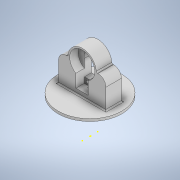
# Autodesk Inventor part: TAPA- 1
Saved by Autodesk Inventor 2021 (Build 250183000, 183)
## iProperties
Created: 2023-04-04
Part Number: TAPA- 1
Material: Generic
Document SubType Name: Modeling
Designer: PC
Density: 1 g/cm^3
Appearance: Default
Author: PC
Autodesk Inventor part; units mm, degrees
ref_plane "YZ Plane" through (0, 0, 0) normal (1, 0, 0) x (0, 1, 0)
ref_plane "XZ Plane" through (0, 0, 0) normal (0, 1, 0) x (-1, 0, 0)
sketch "Sketch1" plane through (0, 0, 0) normal (0, 1, 0) x (-1, 0, 0)
  point P0 (0, 0)
ref_plane "Work Plane26" through (0, 4, 0) normal (0, 1, 0) x (1, 0, 0)
ref_plane "Work Plane42" through (0, 54.25, 0) normal (0, 1, 0) x (-1, 0, 0)
sketch "Sketch7" plane through (0, 54.25, 0) normal (0, 1, 0) x (-1, 0, 0)
  circle A0 centre (0, 0) radius 50 projected
  circle A1 centre (0, 0) radius 52.5
  dimension "d12" = 105
  constraints: 1 centre point, 1 coincident
  measures "d12" diameter of A1
extrude "Extrusion5" add sketch "Sketch7" along normal blind 4 contours A0 | A1
ref_plane "Work Plane34" through (0, 58.25, 0) normal (0, 1, 0) x (1, 0, 0)
sketch "Sketch8" plane through (0, 58.25, 0) normal (0, 1, 0) x (1, 0, 0)
  circle A0 centre (0, 0) radius 51
  dimension "d15" = 102
  constraints: 1 centre point, 1 coincident
  measures "d15" diameter of A0
extrude "Extrusion6" cut sketch "Sketch8" against normal blind 4.5
ref_plane "Work Plane33" through (0, 58.25, 0) normal (0, 1, 0) x (1, 0, 0)
sketch "Sketch12" plane through (0, 58.25, 0) normal (0, 1, 0) x (1, 0, 0)
  circle A0 centre (0, 0) radius 52.5
  constraints: 1 centre point, 1 coincident
extrude "Extrusion7" add sketch "Sketch12" along normal blind 4
ref_plane "Work Plane30" through (0, 54.25, 0) normal (0, 1, 0) x (-1, 0, 0)
sketch "Sketch10" plane through (0, 54.25, 0) normal (0, 1, 0) x (-1, 0, 0)
  point P0 (0, 0)
ref_plane "Work Plane31" through (0, 54.25, 0) normal (0, 1, 0) x (-1, 0, 0)
sketch "Sketch11" plane through (0, 54.25, 0) normal (0, 1, 0) x (-1, 0, 0)
  point P0 (0, 0)
sketch "Sketch13" plane through (0, 62.25, 0) normal (0, 1, 0) x (1, 0, 0)
  point P0 (0, 0)
ref_plane "Work Plane35" through (0, 62.25, 0) normal (0, 1, 0) x (1, 0, 0)
sketch "Sketch18" plane through (0, 0, 0) normal (0, 1, 0) x (-1, 0, 0)
  point P0 (0, 0)
sketch "Sketch19" plane through (0, 0, 0) normal (0, 0, 1) x (1, 0, 0)
  point P0 (0, 0)
sketch "Sketch32" plane through (0, 62.25, 0) normal (0, 1, 0) x (1, 0, 0)
  point P0 (0, 0)
sketch "Sketch33" plane through (0, 62.25, 0) normal (0, 1, 0) x (1, 0, 0)
  point P0 (0, 0)
sketch "Sketch34" plane through (0, 62.25, 0) normal (0, 1, 0) x (1, 0, 0)
  point P0 (0, 0)
sketch "Sketch35" plane through (0, 62.25, 0) normal (0, 1, 0) x (1, 0, 0)
  point P0 (0, 0)
ref_plane "Work Plane3" through (0, 0, 0) normal (0, 0, 1) x (1, 0, 0)
sketch "Sketch55" plane through (0, 62.25, 0) normal (0, 1, 0) x (1, 0, 0)
  line L0 (-39.0297, 12.7817) -> (39.0297, 12.7817)
  line L1 (39.0297, 12.7817) -> (39.0297, -12.7817)
  line L2 (39.0297, -12.7817) -> (-39.0297, -12.7817)
  line L3 (-39.0297, -12.7817) -> (-39.0297, 12.7817)
  circle A0 centre (0, 0) radius 2.55 projected
  line L4 (-39.0297, 12.7817) -> (39.0297, -12.7817) construction
  line L5 (39.0297, 12.7817) -> (-39.0297, -12.7817) construction
  constraints: 12 end point, 2 midpoint, 2 parallel, 1 horizontal, 1 perpendicular
extrude "Extrusion27" add sketch "Sketch55" along normal blind 46.75 contours L0 L1 L2 L3 | A0
ref_plane "Work Plane41" through (-39.0297, 62.25, 12.7817) normal (0, 0, 1) x (1, 0, 0)
sketch "Sketch56" plane through (-39.0297, 62.25, 12.7817) normal (0, 0, 1) x (1, 0, 0)
  line L0 (0, 46.75) -> (78.0595, 46.75) projected
  circle A0 centre (39.0297, 46.75) radius 23.1991
  point P0 (39.0297, -62.25)
  constraints: 1 centre point, 1 midpoint
extrude "Extrusion28" add sketch "Sketch56" against normal blind 25.5634
sketch "Sketch57" plane through (-39.0297, 62.25, 12.7817) normal (0, 0, 1) x (1, 0, 0)
  point P0 (39.0297, -62.25)
sketch "Sketch58" plane through (-39.0297, 62.25, 12.7817) normal (0, 0, 1) x (1, 0, 0)
  point P0 (39.0297, -62.25)
sketch "Sketch59" plane through (-39.0297, 62.25, 12.7817) normal (0, 0, 1) x (1, 0, 0)
  point P0 (39.0297, -62.25)
sketch "Sketch60" plane through (-39.0297, 62.25, 12.7817) normal (0, 0, 1) x (1, 0, 0)
  arc A0 (62.2289, 46.75) -> (15.8306, 46.75) centre (39.0297, 46.75) ccw projected
  circle A1 centre (39.0297, 46.75) radius 10.5
  point P0 (39.0297, -62.25)
  dimension "d99" = 21
  constraints: 1 centre point, 1 coincident
  measures "d99" diameter of A1
sketch "Sketch61" plane through (-39.0297, 62.25, 12.7817) normal (0, 0, 1) x (1, 0, 0)
  point P0 (39.0297, -62.25)
sketch "Sketch62" plane through (-39.0297, 62.25, 12.7817) normal (0, 0, 1) x (1, 0, 0)
  line L0 (29.0297, 16.4771) -> (49.0297, 16.4771)
  line L1 (49.0297, 16.4771) -> (49.0297, 57.4771)
  line L2 (49.0297, 57.4771) -> (29.0297, 57.4771)
  line L3 (29.0297, 57.4771) -> (29.0297, 16.4771)
  line L4 (29.0297, 16.4771) -> (49.0297, 57.4771) construction
  line L5 (49.0297, 16.4771) -> (29.0297, 57.4771) construction
  point P0 (39.0297, -62.25)
  point P1 (39.0297, 36.9771)
  dimension "d102" = 20
  dimension "d103" = 41
  constraints: 12 end point, 2 midpoint, 2 parallel, 1 horizontal, 1 perpendicular
  measures "d102" distance of L2.end L1.end
  measures "d103" distance of L1.end L0.end
extrude "Extrusion30" cut sketch "Sketch62" against normal blind 11.995
sketch "Sketch63" plane through (0, 0, 0) normal (0, 0, 1) x (1, 0, 0)
  point P0 (0, 0)
extrude "Extrusion29" cut sketch "Sketch60" against normal blind 41.495
sketch "Sketch64" plane through (0, 0, 0) normal (0, 0, 1) x (1, 0, 0)
  point P0 (0, 0)
ref_plane "Work Plane4" through (0, 4, -50) normal (0, 0, -1) x (-1, 0, 0)
ref_plane "Work Plane40" through (-39.0297, 62.25, 12.7817) normal (0, 0, 1) x (1, 0, 0)
sketch "Sketch68" plane through (-39.0297, 62.25, 12.7817) normal (0, 0, 1) x (1, 0, 0)
  line L0 (29.0297, 57.4771) -> (49.0297, 57.4771) projected
  line L1 (29.0297, 57.4771) -> (49.0297, 57.4771)
  line L2 (49.0297, 57.4771) -> (49.0297, 64.1771)
  line L3 (49.0297, 64.1771) -> (29.0297, 64.1771)
  line L4 (29.0297, 64.1771) -> (29.0297, 57.4771)
  line L5 (49.0297, 16.4771) -> (29.0297, 16.4771) projected
  line L6 (29.0297, 16.4771) -> (49.0297, 16.4771)
  line L7 (49.0297, 16.4771) -> (49.0297, 9.7771)
  line L8 (49.0297, 9.7771) -> (29.0297, 9.7771)
  line L9 (29.0297, 9.7771) -> (29.0297, 16.4771)
  point P0 (39.0297, -62.25)
  dimension "d110" = 6.7
  dimension "d111" = 6.7
  constraints: 16 end point, 5 equal length, 2 perpendicular, 1 horizontal
  measures "d110" distance of L2.end L0.end
  measures "d111" distance of L5.start L7.end
sketch "Sketch69" plane through (-39.0297, 62.25, 12.7817) normal (0, 0, 1) x (1, 0, 0)
  point P0 (39.0297, -62.25)
sketch "Sketch70" plane through (-39.0297, 62.25, 12.7817) normal (0, 0, 1) x (1, 0, 0)
  point P0 (39.0297, -62.25)
sketch "Sketch71" plane through (-39.0297, 62.25, 12.7817) normal (0, 0, 1) x (1, 0, 0)
  line L0 (28.9579, 61.806) -> (38.9579, 61.806)
  line L1 (38.9579, 61.806) -> (48.9579, 61.806)
  circle A0 centre (33.9579, 61.806) radius 2.5
  circle A1 centre (43.9579, 61.806) radius 2.5
  point P0 (39.0297, -62.25)
  dimension "d112" = 10
  dimension "d113" = 10
  dimension "d114" = 5
  dimension "d115" = 5
  constraints: 4 end point, 3 midpoint, 2 centre point, 1 horizontal, 1 point on line
  measures "d112" distance of L0.start L0.end
  measures "d113" distance of L0.end L1.end
  measures "d114" diameter of A0
  measures "d115" diameter of A1
sketch "Sketch72" plane through (-39.0297, 62.25, 12.7817) normal (0, 0, 1) x (1, 0, 0)
  point P0 (39.0297, -62.25)
extrude "Extrusion33" cut sketch "Sketch71" against normal blind 29
sketch "Sketch73" plane through (-39.0297, 62.25, 12.7817) normal (0, 0, 1) x (1, 0, 0)
  point P0 (39.0297, -62.25)
sketch "Sketch75" plane through (-39.0297, 62.25, 12.7817) normal (0, 0, 1) x (1, 0, 0)
  line L0 (28.9566, 12.0209) -> (38.9566, 12.0209)
  line L1 (38.9566, 12.0209) -> (48.9566, 12.0209)
  circle A0 centre (33.9566, 12.0209) radius 2.5
  circle A1 centre (43.9566, 12.0209) radius 2.5
  point P0 (39.0297, -62.25)
  dimension "d118" = 10
  dimension "d119" = 10
  dimension "d120" = 5
  dimension "d121" = 5
  constraints: 4 end point, 2 centre point, 2 midpoint, 1 horizontal, 1 point on line
  measures "d118" distance of L0.start L0.end
  measures "d119" distance of L0.end L1.end
  measures "d120" diameter of A0
  measures "d121" diameter of A1
extrude "Extrusion34" cut sketch "Sketch75" against normal blind 41.75
fillet "Fillet8" radius 13 1 edges at (-39.0297, 109, 0)
fillet "Fillet9" radius 13 1 edges at (39.0297, 109, 0)
sketch "Sketch134" plane through (0, 58.25, 0) normal (0, -1, 0) x (1, 0, 0)
  circle A0 centre (0, 0) radius 2.5
  dimension "d272" = 5
  constraints: 1 centre point, 1 coincident
  measures "d272" diameter of A0
extrude "Extrusion64" cut sketch "Sketch134" against normal blind 14
sketch "Sketch135" plane through (0, 58.25, 0) normal (0, -1, 0) x (1, 0, 0)
  point P0 (0, 0)
sketch "Sketch136" plane through (0, 58.25, 0) normal (0, -1, 0) x (1, 0, 0)
  point P0 (0, 0)
sketch "Sketch137" plane through (0, 58.25, 0) normal (0, -1, 0) x (1, 0, 0)
  circle A0 centre (0, 0) radius 52.5
  constraints: 1 centre point, 1 coincident
extrude "Extrusion65" cut sketch "Sketch137" along normal blind 10.25
sketch "Sketch140" plane through (-39.0297, 62.25, 12.7817) normal (0, 0, 1) x (1, 0, 0)
  arc A0 (49.0297, 49.9516) -> (29.0297, 49.9516) centre (39.0297, 46.75) ccw projected
  circle A1 centre (39.0297, 46.75) radius 20.665
  line L0 (29.0297, 49.9516) -> (29.0297, 57.4771) projected
  line L1 (29.0297, 57.4771) -> (49.0297, 57.4771)
  line L2 (49.0297, 57.4771) -> (49.0297, 7.5135)
  line L3 (49.0297, 7.5135) -> (29.0297, 7.5135)
  line L4 (29.0297, 7.5135) -> (29.0297, 57.4771)
  point P0 (39.0297, -62.25)
  point P1 (49.0297, 28.6657)
  point P2 (29.0297, 28.6657)
  constraints: 8 end point, 2 parallel, 1 centre point, 1 coincident, 1 horizontal, 1 perpendicular
extrude "Extrusion68" cut sketch "Sketch140" against normal blind 14
sketch "Sketch142" plane through (-39.0297, 62.25, -1.2183) normal (0, 0, 1) x (1, 0, 0)
  line L0 (49.0297, 28.6657) -> (49.0297, 7.5135) projected
  line L1 (28.5297, 57.25) -> (49.0297, 57.25)
  line L2 (49.0297, 57.25) -> (49.0297, 18.0896)
  line L3 (49.0297, 18.0896) -> (28.5297, 18.0896)
  line L4 (28.5297, 18.0896) -> (28.5297, 57.25)
  point P0 (39.0297, -62.25)
  constraints: 8 end point, 2 parallel, 1 horizontal, 1 midpoint, 1 perpendicular
extrude "Extrusion69" cut sketch "Sketch142" against normal blind 14
sketch "Sketch143" plane through (-39.0297, 62.25, 12.7817) normal (0, 0, 1) x (1, 0, 0)
  arc A0 (49.0297, 43.5484) -> (49.0297, 49.9516) centre (39.0297, 46.75) ccw projected
  circle A1 centre (39.0297, 46.75) radius 11.1151
  point P0 (39.0297, -62.25)
  constraints: 1 centre point, 1 coincident
extrude "Extrusion70" cut sketch "Sketch143" against normal blind 40.5
sketch "Sketch144" plane through (-39.0297, 62.25, -1.2183) normal (0, 0, 1) x (1, 0, 0)
  arc A0 (28.5297, 28.9513) -> (29.0297, 28.6657) centre (39.0297, 46.75) ccw projected
  line L0 (28.5297, 18.0896) -> (29.0297, 18.0896) projected
  line L1 (29.0297, 28.6657) -> (28.5297, 28.6657)
  line L2 (28.5297, 28.6657) -> (28.5297, 18.0896)
  line L3 (28.5297, 18.0896) -> (29.0297, 18.0896)
  line L4 (29.0297, 18.0896) -> (29.0297, 28.6657)
  point P0 (39.0297, -62.25)
  constraints: 8 end point, 2 parallel, 1 horizontal, 1 perpendicular
extrude "Extrusion71" cut sketch "Sketch144" along normal blind 40.5 and the other way blind 20.25
sketch "Sketch145" plane through (-39.0297, 62.25, 12.7817) normal (0, 0, 1) x (1, 0, 0)
  arc A0 (28.5297, 28.9513) -> (29.0297, 28.6657) centre (39.0297, 46.75) ccw projected
  line L0 (28.5297, 43.1036) -> (28.5297, 26.0631) projected
  line L1 (29.0297, 28.6657) -> (28.5297, 28.6657)
  line L2 (28.5297, 28.6657) -> (28.5297, 28.9897)
  line L3 (28.5297, 28.9897) -> (29.0297, 28.9897)
  line L4 (29.0297, 28.9897) -> (29.0297, 28.6657)
  point P0 (39.0297, -62.25)
  constraints: 8 end point, 2 parallel, 1 horizontal, 1 perpendicular, 1 point on line
extrude "Extrusion72" cut sketch "Sketch145" against normal blind 40.5
sketch "Sketch147" plane through (-39.0297, 62.25, -1.2183) normal (0, 0, 1) x (1, 0, 0)
  line L0 (28.5297, 50.3964) -> (28.5297, 57.25) projected
  line L1 (49.0297, 18.0896) -> (49.0297, 7.5135) projected
  line L2 (28.5297, 57.25) -> (49.0297, 57.25)
  line L3 (49.0297, 57.25) -> (49.0297, 7.5135)
  line L4 (49.0297, 7.5135) -> (28.5297, 7.5135)
  line L5 (28.5297, 7.5135) -> (28.5297, 57.25)
  point P0 (39.0297, -62.25)
  constraints: 8 end point, 2 parallel, 1 horizontal, 1 perpendicular
extrude "Extrusion73" cut sketch "Sketch147" along normal blind 21.75
sketch "Sketch148" plane through (-39.0297, 62.25, -1.2183) normal (0, 0, 1) x (1, 0, 0)
  line L0 (35.3834, 57.25) -> (28.5297, 57.25) projected
  line L1 (49.0297, 28.6657) -> (49.0297, 7.5135) projected
  line L2 (28.5297, 57.25) -> (49.0297, 57.25)
  line L3 (49.0297, 57.25) -> (49.0297, 16.75)
  line L4 (49.0297, 16.75) -> (28.5297, 16.75)
  line L5 (28.5297, 16.75) -> (28.5297, 57.25)
  point P0 (39.0297, -62.25)
  dimension "d297" = 40.5
  constraints: 8 end point, 2 parallel, 1 horizontal, 1 perpendicular, 1 point on line
  measures "d297" distance of L2.end L3.end
extrude "Extrusion74" cut sketch "Sketch148" against normal blind 21.75
fillet "Fillet10" radius 2 4 edges at (0, 62.25, 12.7817) (39.0297, 62.25, 0) (0, 62.25, -12.7817) (-39.0297, 62.25, 0)
fillet "Fillet11" radius 2 2 edges at (-23.1991, 109, 0) (23.1991, 109, 0)
sketch "Sketch149" plane through (-39.0297, 62.25, -12.7817) normal (0, 0, -1) x (-1, 0, 0)
  point P0 (-39.0297, -62.25)
sketch "Sketch150" plane through (-39.0297, 62.25, -12.7817) normal (0, 0, -1) x (-1, 0, 0)
  point P0 (-39.0297, -62.25)
sketch "Sketch151" plane through (0, 58.25, 0) normal (0, -1, 0) x (1, 0, 0)
  circle A0 centre (0, 0) radius 2.6
  dimension "d302" = 5.2
  constraints: 1 centre point, 1 coincident
  measures "d302" diameter of A0
extrude "Extrusion75" cut sketch "Sketch151" against normal blind 14
sketch "Sketch152" plane through (-39.0297, 62.25, -1.2183) normal (0, 0, 1) x (1, 0, 0)
  point P0 (39.0297, -62.25)
sketch "Sketch153" plane through (0, 58.25, 0) normal (0, -1, 0) x (1, 0, 0)
  point P0 (0, 0)
sketch "Sketch154" plane through (0, 58.25, 0) normal (0, -1, 0) x (1, 0, 0)
  point P0 (0, 0)
sketch "Sketch155" plane through (0, 58.25, 0) normal (0, -1, 0) x (1, 0, 0)
  circle A0 centre (0, 0) radius 2.6
  constraints: 1 centre point, 1 coincident
extrude "Extrusion76" add sketch "Sketch155" against normal blind 14.5
sketch "Sketch156" plane through (-39.0297, 64.25, 12.7817) normal (0, 0, 1) x (1, 0, 0)
  line L0 (28.5297, 48.3964) -> (28.5297, 55.25) projected
  line L1 (49.0297, 14.75) -> (49.0297, 5.5135) projected
  line L2 (28.5297, 55.25) -> (49.0297, 55.25)
  line L3 (49.0297, 55.25) -> (49.0297, 5.5135)
  line L4 (49.0297, 5.5135) -> (28.5297, 5.5135)
  line L5 (28.5297, 5.5135) -> (28.5297, 55.25)
  point P0 (39.0297, -64.25)
  constraints: 8 end point, 2 parallel, 1 horizontal, 1 perpendicular
extrude "Extrusion77" cut sketch "Sketch156" against normal blind 14
sketch "Sketch157" plane through (0, 62.25, 0) normal (0, 1, 0) x (1, 0, 0)
  point P0 (0, 0)
sketch "Sketch158" plane through (0, 58.25, 0) normal (0, -1, 0) x (1, 0, 0)
  circle A0 centre (0, 0) radius 2.75
  line L0 (-2.75, 0) -> (1.85, 0)
  line L1 (1.85, 0) -> (1.85, 2.0347)
  line L2 (1.85, 0) -> (1.85, -2.0347)
  dimension "d309" = 5.5
  dimension "d310" = 4.6
  constraints: 6 end point, 3 point on circle, 2 vertical, 1 centre point, 1 coincident, 1 horizontal
  measures "d309" diameter of A0
  measures "d310" distance of L0.start L0.end
extrude "Extrusion78" cut sketch "Sketch158" against normal blind 14 contours L1 L0 A0 | A0 L0 L2
sketch "Sketch159" plane through (-39.0297, 64.25, 12.7817) normal (0, 0, 1) x (1, 0, 0)
  point P0 (39.0297, -64.25)
sketch "Sketch160" plane through (0, 58.25, 0) normal (0, -1, 0) x (1, 0, 0)
  circle A0 centre (0, 0) radius 2.75
  constraints: 1 centre point, 1 coincident
extrude "Extrusion79" add sketch "Sketch160" against normal blind 14
sketch "Sketch161" plane through (-39.0297, 64.25, 12.7817) normal (0, 0, 1) x (1, 0, 0)
  line L0 (28.5297, 48.3964) -> (28.5297, 55.25) projected
  line L1 (49.0297, 14.75) -> (49.0297, 5.5135) projected
  line L2 (28.5297, 55.25) -> (49.0297, 55.25)
  line L3 (49.0297, 55.25) -> (49.0297, 5.5135)
  line L4 (49.0297, 5.5135) -> (28.5297, 5.5135)
  line L5 (28.5297, 5.5135) -> (28.5297, 55.25)
  point P0 (39.0297, -64.25)
  constraints: 8 end point, 2 parallel, 1 horizontal, 1 perpendicular
extrude "Extrusion80" cut sketch "Sketch161" against normal blind 14
sketch "Sketch162" plane through (0, 58.25, 0) normal (0, -1, 0) x (1, 0, 0)
  circle A0 centre (0, 0) radius 2.75
  line L0 (-2.75, 0) -> (2.25, 0)
  line L1 (2.25, 0) -> (2.25, 1.5811)
  line L2 (2.25, 0) -> (2.25, -1.6149)
  line L3 (-3.6464, -1.2183) -> (3.6464, -1.2183) projected
  point P0 (2.25, -1.5811)
  dimension "d317" = 5.5
  dimension "d318" = 5
  constraints: 6 end point, 2 point on circle, 1 centre point, 1 coincident, 1 horizontal, 1 perpendicular, 1 vertical
  measures "d317" diameter of A0
  measures "d318" distance of L0.start L0.end
extrude "Extrusion81" cut sketch "Sketch162" against normal blind 14 contours L1 L0 A0 | L0 L2 L3 A0 | A0 L3 L2 picked at (-0.7794, -1.395)
sketch "Sketch163" plane through (0, 58.25, 0) normal (0, -1, 0) x (1, 0, 0)
  circle A0 centre (0, 0) radius 2.75
  constraints: 1 centre point, 1 coincident
extrude "Extrusion82" add sketch "Sketch163" against normal blind 14.5
sketch "Sketch164" plane through (-39.0297, 64.25, 12.7817) normal (0, 0, 1) x (1, 0, 0)
  line L0 (49.0297, 26.6657) -> (49.0297, 5.5135) projected
  line L1 (35.3834, 55.25) -> (28.5297, 55.25) projected
  line L2 (49.0297, 5.5135) -> (28.5297, 5.5135)
  line L3 (28.5297, 5.5135) -> (28.5297, 55.25)
  line L4 (28.5297, 55.25) -> (49.0297, 55.25)
  line L5 (49.0297, 55.25) -> (49.0297, 5.5135)
  point P0 (39.0297, -64.25)
  constraints: 8 end point, 2 parallel, 1 horizontal, 1 perpendicular
extrude "Extrusion83" cut sketch "Sketch164" against normal blind 14
sketch "Sketch165" plane through (0, 58.25, 0) normal (0, -1, 0) x (1, 0, 0)
  circle A0 centre (0, 0) radius 2.6
  line L0 (-2.6, 0) -> (2.1, 0)
  line L1 (2.1, 0) -> (2.1, 1.533)
  line L2 (2.1, 0) -> (2.1, -1.533)
  dimension "d325" = 5.2
  dimension "d326" = 4.7
  constraints: 6 end point, 3 point on circle, 2 vertical, 1 centre point, 1 coincident, 1 horizontal
  measures "d325" diameter of A0
  measures "d326" distance of L0.start L0.end
extrude "Extrusion84" cut sketch "Sketch165" against normal blind 14 contours L1 L0 A0 | A0 L0 L2
sketch "Sketch166" plane through (0, 58.25, 0) normal (0, -1, 0) x (1, 0, 0)
  point P0 (0, 0)
sketch "Sketch167" plane through (0, 58.25, 0) normal (0, -1, 0) x (1, 0, 0)
  point P0 (0, 0)
body "Solid1"
